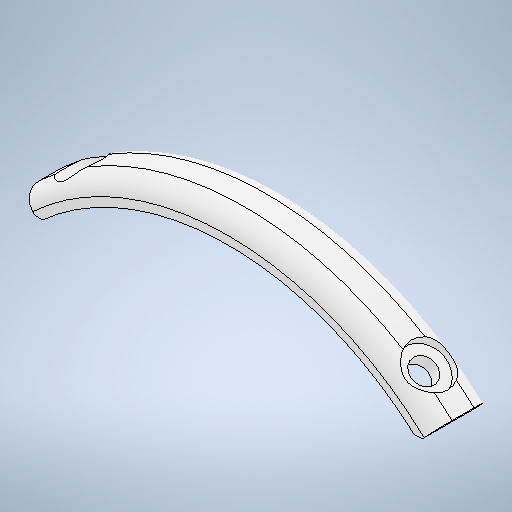
# Autodesk Inventor part: joint4_frame_support_fixture
Saved by Autodesk Inventor 2025.3 (Build 293356030, 356C)
## iProperties
Created: 2025-11-09
Part Number: joint4_frame_support_fixture
Material: PLA filament
Document SubType Name: Modeling
Designer: MSI
Mass: 3.56123 g
Surface Area: 22.3953 cm^2
Volume: 2.96769 cm^3
Density: 1.2 g/cm^3
Appearance: 일반
Author: MSI
Autodesk Inventor part; units mm, degrees
ref_plane "YZ Plane" through (0, 0, 0) normal (1, 0, 0) x (0, 1, 0)
ref_plane "XZ Plane" through (0, 0, 0) normal (0, 1, 0) x (-1, 0, 0)
sketch "스케치1" plane through (0, 0, 0) normal (0, 0, 1) x (1, 0, 0)
  arc A0 (37.5099, 40.2245) -> (-37.5099, 40.2245) centre (0, 0) ccw
  line L0 (-37.5099, 40.2245) -> (0, 0)
  line L1 (0, 0) -> (37.5099, 40.2245)
  line L2 (0, 0) -> (0, 55)
  circle A1 centre (0, 0) radius 50.5
  point P0 (34.4409, 36.9334)
  point P1 (-34.4409, 36.9334)
  dimension "d1" = 55
  dimension "d2" = 43
  dimension "d3" = 43
  dimension "d4" = 4.5
  constraints: 6 end point, 3 point on circle, 2 centre point, 2 coincident, 1 vertical
  measures "d1" radius of A0
  measures "d2" angle of L2 L0
  measures "d3" angle of L2 L1
  measures "d4" radial gap between concentric circles of A0 A1
extrude "돌출1" add sketch "스케치1" along normal mid plane 10 contours L1 A1 L2 A0 | L2 A1 L0 A0
sketch "스케치2" plane through (0, 0, 0) normal (0, 0, 1) x (1, 0, 0)
  line L0 (0, 0) -> (-31.5467, 45.0534)
  arc A0 (37.5099, 40.2245) -> (-37.5099, 40.2245) centre (0, 0) ccw projected
  line L1 (0, 0) -> (0, 40.0964) construction
  dimension "d7" = 35
  constraints: 4 end point, 1 point on circle, 1 vertical
  measures "d7" angle of L0 L1
ref_plane "작업 평면1" through (-31.5467, 45.0534, 0) normal (-0.5735764, 0.819152, 0) x (-0.819152, -0.5735764, 0)
sketch "스케치3" plane through (-31.5467, 45.0534, 0) normal (-0.5735764, 0.819152, 0) x (-0.819152, -0.5735764, 0)
  point P0 (0, 0)
  point P1 (0, 0)
  constraints: 1 coincident
hole "구멍1" at (-31.5467, 45.0534, 0) direction (0.5735764, -0.819152, 0) diameter 4.5 end through all counterbore diameter 8 counterbore depth 2 clearance for "Socket Head Cap Screw ISO 4762" size "M4" standard "ISO"
mirror "미러1" about plane through (0, 0, 0) normal (1, 0, 0) of "구멍1"
fillet "모깎기1" radius 3 2 edges at (0, 55, 5) (0, 55, -5)
chamfer "모따기1" distance 1 angle 45 2 edges at (34.4409, 36.9334, 0) (-34.4409, 36.9334, 0)
equation "\"d3\" = d2"
